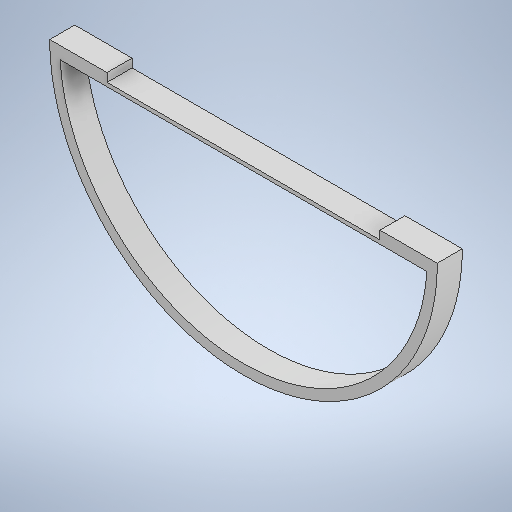
# Autodesk Inventor part: Siding Revised
Saved by Autodesk Inventor 2025 (Build 290162010, 162A)
## iProperties
Created: 2024-06-06
Part Number: Siding Revised
Material: Generic
Document SubType Name: Modeling
Designer: vncnt
Density: 1 g/cm^3
Appearance: Default
Author: vncnt
Autodesk Inventor part; units mm, degrees
ref_plane "YZ Plane" through (0, 0, 0) normal (1, 0, 0) x (0, 1, 0)
ref_plane "XZ Plane" through (0, 0, 0) normal (0, 1, 0) x (-1, 0, 0)
ref_plane "XY Plane" through (0, 0, 0) normal (0, 0, 1) x (1, 0, 0)
sketch "Sketch1" plane through (0, 0, 0) normal (0, 0, 1) x (1, 0, 0)
  arc A0 (37.1972, 10.8951) -> (38.76, 0) centre (0, 0) ccw
  arc A1 (-36.6776, -2.4605) -> (36.6776, -2.4605) centre (0, 0) ccw
  line L0 (-36.76, 0) -> (36.76, 0)
  line L1 (-36.76, 0) -> (37.1972, 0)
  line L2 (36.6776, -2.4605) -> (-36.6776, -2.4605)
  line L3 (-36.76, 0) -> (-38.76, 0)
  line L4 (37.1972, 0) -> (38.76, 0)
  line L5 (0, 0) -> (27.3, 0)
  line L6 (27.3, 0) -> (27.3, -1.7)
  line L7 (27.3, -1.7) -> (0, -1.7)
  line L8 (0, -1.7) -> (0, 0)
  line L9 (-27.3, 0) -> (-27.3, -1.7)
  line L10 (-27.3, -1.7) -> (0, -1.7)
  dimension "d0" = 77.52
  dimension "d1" = 2
  constraints: 22 end point, 5 point on circle, 4 horizontal, 3 parallel, 2 centre point, 2 point on line, 2 symmetric about line, 1 coincident, 1 perpendicular
  measures "d0" diameter of A0
  measures "d1" radial gap between concentric circles of A0 A1
extrude "Extrusion1" add sketch "Sketch1" along normal blind 5 contours L3 L0 L9 L10 L7 L6 L1 L4 A0
body "Solid1"
